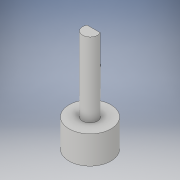
# Autodesk Inventor part: Potentiometer
Saved by Autodesk Inventor 2018 (Build 220112000, 112)
## iProperties
Created: 2017-12-06
Part Number: Potentiometer
Material: Generic
Document SubType Name: Modeling
Designer: Andrew
Density: 1 g/cm^3
Appearance: Default
Author: Andrew
Autodesk Inventor part; units mm, degrees
ref_plane "YZ Plane" through (0, 0, 0) normal (1, 0, 0) x (0, 1, 0)
ref_plane "XZ Plane" through (0, 0, 0) normal (0, 1, 0) x (-1, 0, 0)
ref_plane "XY Plane" through (0, 0, 0) normal (0, 0, 1) x (1, 0, 0)
sketch "Sketch1" plane through (0, 0, 0) normal (0, 1, 0) x (-1, 0, 0)
  circle A0 centre (0, 0) radius 8.382
  circle A1 centre (0, 0) radius 2.9845
  dimension "d0" = 5.969
  dimension "d1" = 16.764
  constraints: 2 centre point, 2 coincident
  measures "d0" diameter of A1
  measures "d1" diameter of A0
extrude "Extrusion1" add sketch "Sketch1" against normal blind 11.176 contours A0 | A1
extrude "Extrusion2" add sketch "Sketch1" along normal blind 29.7942 contours A1
sketch "Sketch2" plane through (0, 29.7942, 0) normal (0, 1, 0) x (1, 0, 0)
  circle A0 centre (0, 0) radius 2.9845 projected
  circle A1 centre (0, 0) radius 2.9845 projected
  line L0 (-2.6027, 1.4605) -> (2.6027, 1.4605)
  arc A2 (2.6027, 1.4605) -> (-2.6027, 1.4605) centre (0, 0) ccw
  dimension "d6" = 4.445
  constraints: 4 point on circle, 2 end point, 1 centre point, 1 concentric, 1 horizontal
extrude "Extrusion3" cut sketch "Sketch2" against normal blind 11.8872 contours L0 A0 picked at (-0.1168, 1.9616)
body "Solid1"
